Autodesk Inventor part; units mm, degrees
(part 2 of 5)
  line L926 (78.7001, 18.8118) -> (79.4901, 18.8118)
  line L927 (79.4901, 18.8118) -> (79.4901, 18.4118)
  line L928 (78.6251, 11.5368) -> (77.0251, 11.5368)
  line L929 (77.0251, 11.5368) -> (77.0251, 12.1868)
  line L930 (77.0251, 12.1868) -> (78.6251, 12.1868)
  line L931 (78.6251, 12.1868) -> (78.6251, 11.5368)
  line L932 (78.6251, 19.4368) -> (77.0251, 19.4368)
  line L933 (77.0251, 19.4368) -> (77.0251, 20.0868)
  line L934 (77.0251, 20.0868) -> (78.6251, 20.0868)
  line L935 (78.6251, 20.0868) -> (78.6251, 19.4368)
  line L936 (41.1326, 37.3618) -> (41.9226, 37.3618)
  line L937 (41.9226, 37.3618) -> (41.9226, 36.9618)
  line L938 (41.9226, 36.9618) -> (41.1326, 36.9618)
  line L939 (41.1326, 36.9618) -> (41.1326, 37.3618)
  line L940 (38.5926, 37.3618) -> (39.3826, 37.3618)
  line L941 (39.3826, 37.3618) -> (39.3826, 36.9618)
  line L942 (39.3826, 36.9618) -> (38.5926, 36.9618)
  line L943 (38.5926, 36.9618) -> (38.5926, 37.3618)
  line L944 (41.1326, 36.5618) -> (41.9226, 36.5618)
  line L945 (41.9226, 36.5618) -> (41.9226, 36.1618)
  line L946 (41.9226, 36.1618) -> (41.1326, 36.1618)
  line L947 (41.1326, 36.1618) -> (41.1326, 36.5618)
  line L948 (38.5926, 36.5618) -> (39.3826, 36.5618)
  line L949 (39.3826, 36.5618) -> (39.3826, 36.1618)
  line L950 (39.3826, 36.1618) -> (38.5926, 36.1618)
  line L951 (38.5926, 36.1618) -> (38.5926, 36.5618)
  line L952 (41.1326, 35.7618) -> (41.9226, 35.7618)
  line L953 (41.9226, 35.7618) -> (41.9226, 35.3618)
  line L954 (41.9226, 35.3618) -> (41.1326, 35.3618)
  line L955 (41.1326, 35.3618) -> (41.1326, 35.7618)
  line L956 (38.5926, 35.7618) -> (39.3826, 35.7618)
  line L957 (39.3826, 35.7618) -> (39.3826, 35.3618)
  line L958 (39.3826, 35.3618) -> (38.5926, 35.3618)
  line L959 (38.5926, 35.3618) -> (38.5926, 35.7618)
  line L960 (41.1326, 34.9618) -> (41.9226, 34.9618)
  line L961 (41.9226, 34.9618) -> (41.9226, 34.5618)
  line L962 (41.9226, 34.5618) -> (41.1326, 34.5618)
  line L963 (41.1326, 34.5618) -> (41.1326, 34.9618)
  line L964 (38.5926, 34.9618) -> (39.3826, 34.9618)
  line L965 (39.3826, 34.9618) -> (39.3826, 34.5618)
  line L966 (39.3826, 34.5618) -> (38.5926, 34.5618)
  line L967 (38.5926, 34.5618) -> (38.5926, 34.9618)
  line L968 (41.1326, 34.1618) -> (41.9226, 34.1618)
  line L969 (41.9226, 34.1618) -> (41.9226, 33.7618)
  line L970 (41.9226, 33.7618) -> (41.1326, 33.7618)
  line L971 (41.1326, 33.7618) -> (41.1326, 34.1618)
  line L972 (38.5926, 34.1618) -> (39.3826, 34.1618)
  line L973 (39.3826, 34.1618) -> (39.3826, 33.7618)
  line L974 (39.3826, 33.7618) -> (38.5926, 33.7618)
  line L975 (38.5926, 33.7618) -> (38.5926, 34.1618)
  line L976 (41.1326, 33.3618) -> (41.9226, 33.3618)
  line L977 (41.9226, 33.3618) -> (41.9226, 32.9618)
  line L978 (41.9226, 32.9618) -> (41.1326, 32.9618)
  line L979 (41.1326, 32.9618) -> (41.1326, 33.3618)
  line L980 (38.5926, 33.3618) -> (39.3826, 33.3618)
  line L981 (39.3826, 33.3618) -> (39.3826, 32.9618)
  line L982 (39.3826, 32.9618) -> (38.5926, 32.9618)
  line L983 (38.5926, 32.9618) -> (38.5926, 33.3618)
  line L984 (41.1326, 32.5618) -> (41.9226, 32.5618)
  line L985 (41.9226, 32.5618) -> (41.9226, 32.1618)
  line L986 (41.9226, 32.1618) -> (41.1326, 32.1618)
  line L987 (41.1326, 32.1618) -> (41.1326, 32.5618)
  line L988 (38.5926, 32.5618) -> (39.3826, 32.5618)
  line L989 (39.3826, 32.5618) -> (39.3826, 32.1618)
  line L990 (39.3826, 32.1618) -> (38.5926, 32.1618)
  line L991 (38.5926, 32.1618) -> (38.5926, 32.5618)
  line L992 (41.1326, 31.7618) -> (41.9226, 31.7618)
  line L993 (41.9226, 31.7618) -> (41.9226, 31.3618)
  line L994 (41.9226, 31.3618) -> (41.1326, 31.3618)
  line L995 (41.1326, 31.3618) -> (41.1326, 31.7618)
  line L996 (38.5926, 31.7618) -> (39.3826, 31.7618)
  line L997 (39.3826, 31.7618) -> (39.3826, 31.3618)
  line L998 (39.3826, 31.3618) -> (38.5926, 31.3618)
  line L999 (38.5926, 31.3618) -> (38.5926, 31.7618)
  line L1000 (39.4576, 38.6368) -> (41.0576, 38.6368)
  line L1001 (41.0576, 38.6368) -> (41.0576, 37.9868)
  line L1002 (41.0576, 37.9868) -> (39.4576, 37.9868)
  line L1003 (39.4576, 37.9868) -> (39.4576, 38.6368)
  line L1004 (39.4576, 30.7368) -> (41.0576, 30.7368)
  line L1005 (41.0576, 30.7368) -> (41.0576, 30.0868)
  line L1006 (41.0576, 30.0868) -> (39.4576, 30.0868)
  line L1007 (39.4576, 30.0868) -> (39.4576, 30.7368)
  line L1008 (116.3201, 75.0868) -> (117.1101, 75.0868)
  line L1009 (117.1101, 75.0868) -> (117.1101, 74.6868)
  line L1010 (117.1101, 74.6868) -> (116.3201, 74.6868)
  line L1011 (116.3201, 74.6868) -> (116.3201, 75.0868)
  line L1012 (113.7801, 75.0868) -> (114.5701, 75.0868)
  line L1013 (114.5701, 75.0868) -> (114.5701, 74.6868)
  line L1014 (114.5701, 74.6868) -> (113.7801, 74.6868)
  line L1015 (113.7801, 74.6868) -> (113.7801, 75.0868)
  line L1016 (116.3201, 74.2868) -> (117.1101, 74.2868)
  line L1017 (117.1101, 74.2868) -> (117.1101, 73.8868)
  line L1018 (117.1101, 73.8868) -> (116.3201, 73.8868)
  line L1019 (116.3201, 73.8868) -> (116.3201, 74.2868)
  line L1020 (113.7801, 74.2868) -> (114.5701, 74.2868)
  line L1021 (114.5701, 74.2868) -> (114.5701, 73.8868)
  line L1022 (114.5701, 73.8868) -> (113.7801, 73.8868)
  line L1023 (113.7801, 73.8868) -> (113.7801, 74.2868)
  line L1024 (116.3201, 73.4868) -> (117.1101, 73.4868)
  line L1025 (117.1101, 73.4868) -> (117.1101, 73.0868)
  line L1026 (117.1101, 73.0868) -> (116.3201, 73.0868)
  line L1027 (116.3201, 73.0868) -> (116.3201, 73.4868)
  line L1028 (113.7801, 73.4868) -> (114.5701, 73.4868)
  line L1029 (114.5701, 73.4868) -> (114.5701, 73.0868)
  line L1030 (114.5701, 73.0868) -> (113.7801, 73.0868)
  line L1031 (113.7801, 73.0868) -> (113.7801, 73.4868)
  line L1032 (116.3201, 72.6868) -> (117.1101, 72.6868)
  line L1033 (117.1101, 72.6868) -> (117.1101, 72.2868)
  line L1034 (117.1101, 72.2868) -> (116.3201, 72.2868)
  line L1035 (116.3201, 72.2868) -> (116.3201, 72.6868)
  line L1036 (113.7801, 72.6868) -> (114.5701, 72.6868)
  line L1037 (114.5701, 72.6868) -> (114.5701, 72.2868)
  line L1038 (114.5701, 72.2868) -> (113.7801, 72.2868)
  line L1039 (113.7801, 72.2868) -> (113.7801, 72.6868)
  line L1040 (116.3201, 71.8868) -> (117.1101, 71.8868)
  line L1041 (117.1101, 71.8868) -> (117.1101, 71.4868)
  line L1042 (117.1101, 71.4868) -> (116.3201, 71.4868)
  line L1043 (116.3201, 71.4868) -> (116.3201, 71.8868)
  line L1044 (113.7801, 71.8868) -> (114.5701, 71.8868)
  line L1045 (114.5701, 71.8868) -> (114.5701, 71.4868)
  line L1046 (114.5701, 71.4868) -> (113.7801, 71.4868)
  line L1047 (113.7801, 71.4868) -> (113.7801, 71.8868)
  line L1048 (116.3201, 71.0868) -> (117.1101, 71.0868)
  line L1049 (117.1101, 71.0868) -> (117.1101, 70.6868)
  line L1050 (117.1101, 70.6868) -> (116.3201, 70.6868)
  line L1051 (116.3201, 70.6868) -> (116.3201, 71.0868)
  line L1052 (113.7801, 71.0868) -> (114.5701, 71.0868)
  line L1053 (114.5701, 71.0868) -> (114.5701, 70.6868)
  line L1054 (114.5701, 70.6868) -> (113.7801, 70.6868)
  line L1055 (113.7801, 70.6868) -> (113.7801, 71.0868)
  line L1056 (116.3201, 70.2868) -> (117.1101, 70.2868)
  line L1057 (117.1101, 70.2868) -> (117.1101, 69.8868)
  line L1058 (117.1101, 69.8868) -> (116.3201, 69.8868)
  line L1059 (116.3201, 69.8868) -> (116.3201, 70.2868)
  line L1060 (113.7801, 70.2868) -> (114.5701, 70.2868)
  line L1061 (114.5701, 70.2868) -> (114.5701, 69.8868)
  line L1062 (114.5701, 69.8868) -> (113.7801, 69.8868)
  line L1063 (113.7801, 69.8868) -> (113.7801, 70.2868)
  line L1064 (116.3201, 69.4868) -> (117.1101, 69.4868)
  line L1065 (117.1101, 69.4868) -> (117.1101, 69.0868)
  line L1066 (117.1101, 69.0868) -> (116.3201, 69.0868)
  line L1067 (116.3201, 69.0868) -> (116.3201, 69.4868)
  line L1068 (113.7801, 69.4868) -> (114.5701, 69.4868)
  line L1069 (114.5701, 69.4868) -> (114.5701, 69.0868)
  line L1070 (114.5701, 69.0868) -> (113.7801, 69.0868)
  line L1071 (113.7801, 69.0868) -> (113.7801, 69.4868)
  line L1072 (114.6451, 76.3618) -> (116.2451, 76.3618)
  line L1073 (116.2451, 76.3618) -> (116.2451, 75.7118)
  line L1074 (116.2451, 75.7118) -> (114.6451, 75.7118)
  line L1075 (114.6451, 75.7118) -> (114.6451, 76.3618)
  line L1076 (114.6451, 68.4618) -> (116.2451, 68.4618)
  line L1077 (116.2451, 68.4618) -> (116.2451, 67.8118)
  line L1078 (116.2451, 67.8118) -> (114.6451, 67.8118)
  line L1079 (114.6451, 67.8118) -> (114.6451, 68.4618)
  line L1080 (97.5651, 75.1118) -> (98.3551, 75.1118)
  line L1081 (98.3551, 75.1118) -> (98.3551, 74.7118)
  line L1082 (98.3551, 74.7118) -> (97.5651, 74.7118)
  line L1083 (97.5651, 74.7118) -> (97.5651, 75.1118)
  line L1084 (95.0251, 75.1118) -> (95.8151, 75.1118)
  line L1085 (95.8151, 75.1118) -> (95.8151, 74.7118)
  line L1086 (95.8151, 74.7118) -> (95.0251, 74.7118)
  line L1087 (95.0251, 74.7118) -> (95.0251, 75.1118)
  line L1088 (97.5651, 74.3118) -> (98.3551, 74.3118)
  line L1089 (98.3551, 74.3118) -> (98.3551, 73.9118)
  line L1090 (98.3551, 73.9118) -> (97.5651, 73.9118)
  line L1091 (97.5651, 73.9118) -> (97.5651, 74.3118)
  line L1092 (95.0251, 74.3118) -> (95.8151, 74.3118)
  line L1093 (95.8151, 74.3118) -> (95.8151, 73.9118)
  line L1094 (95.8151, 73.9118) -> (95.0251, 73.9118)
  line L1095 (95.0251, 73.9118) -> (95.0251, 74.3118)
  line L1096 (97.5651, 73.5118) -> (98.3551, 73.5118)
  line L1097 (98.3551, 73.5118) -> (98.3551, 73.1118)
  line L1098 (98.3551, 73.1118) -> (97.5651, 73.1118)
  line L1099 (97.5651, 73.1118) -> (97.5651, 73.5118)
  line L1100 (95.0251, 73.5118) -> (95.8151, 73.5118)
  line L1101 (95.8151, 73.5118) -> (95.8151, 73.1118)
  line L1102 (95.8151, 73.1118) -> (95.0251, 73.1118)
  line L1103 (95.0251, 73.1118) -> (95.0251, 73.5118)
  line L1104 (97.5651, 72.7118) -> (98.3551, 72.7118)
  line L1105 (98.3551, 72.7118) -> (98.3551, 72.3118)
  line L1106 (98.3551, 72.3118) -> (97.5651, 72.3118)
  line L1107 (97.5651, 72.3118) -> (97.5651, 72.7118)
  line L1108 (95.0251, 72.7118) -> (95.8151, 72.7118)
  line L1109 (95.8151, 72.7118) -> (95.8151, 72.3118)
  line L1110 (95.8151, 72.3118) -> (95.0251, 72.3118)
  line L1111 (95.0251, 72.3118) -> (95.0251, 72.7118)
  line L1112 (97.5651, 71.9118) -> (98.3551, 71.9118)
  line L1113 (98.3551, 71.9118) -> (98.3551, 71.5118)
  line L1114 (98.3551, 71.5118) -> (97.5651, 71.5118)
  line L1115 (97.5651, 71.5118) -> (97.5651, 71.9118)
  line L1116 (95.0251, 71.9118) -> (95.8151, 71.9118)
  line L1117 (95.8151, 71.9118) -> (95.8151, 71.5118)
  line L1118 (95.8151, 71.5118) -> (95.0251, 71.5118)
  line L1119 (95.0251, 71.5118) -> (95.0251, 71.9118)
  line L1120 (97.5651, 71.1118) -> (98.3551, 71.1118)
  line L1121 (98.3551, 71.1118) -> (98.3551, 70.7118)
  line L1122 (98.3551, 70.7118) -> (97.5651, 70.7118)
  line L1123 (97.5651, 70.7118) -> (97.5651, 71.1118)
  line L1124 (95.0251, 71.1118) -> (95.8151, 71.1118)
  line L1125 (95.8151, 71.1118) -> (95.8151, 70.7118)
  line L1126 (95.8151, 70.7118) -> (95.0251, 70.7118)
  line L1127 (95.0251, 70.7118) -> (95.0251, 71.1118)
  line L1128 (97.5651, 70.3118) -> (98.3551, 70.3118)
  line L1129 (98.3551, 70.3118) -> (98.3551, 69.9118)
  line L1130 (98.3551, 69.9118) -> (97.5651, 69.9118)
  line L1131 (97.5651, 69.9118) -> (97.5651, 70.3118)
  line L1132 (95.0251, 70.3118) -> (95.8151, 70.3118)
  line L1133 (95.8151, 70.3118) -> (95.8151, 69.9118)
  line L1134 (95.8151, 69.9118) -> (95.0251, 69.9118)
  line L1135 (95.0251, 69.9118) -> (95.0251, 70.3118)
  line L1136 (97.5651, 69.5118) -> (98.3551, 69.5118)
  line L1137 (98.3551, 69.5118) -> (98.3551, 69.1118)
  line L1138 (98.3551, 69.1118) -> (97.5651, 69.1118)
  line L1139 (97.5651, 69.1118) -> (97.5651, 69.5118)
  line L1140 (95.0251, 69.5118) -> (95.8151, 69.5118)
  line L1141 (95.8151, 69.5118) -> (95.8151, 69.1118)
  line L1142 (95.8151, 69.1118) -> (95.0251, 69.1118)
  line L1143 (95.0251, 69.1118) -> (95.0251, 69.5118)
  line L1144 (95.8901, 76.3868) -> (97.4901, 76.3868)
  line L1145 (97.4901, 76.3868) -> (97.4901, 75.7368)
  line L1146 (97.4901, 75.7368) -> (95.8901, 75.7368)
  line L1147 (95.8901, 75.7368) -> (95.8901, 76.3868)
  line L1148 (95.8901, 68.4868) -> (97.4901, 68.4868)
  line L1149 (97.4901, 68.4868) -> (97.4901, 67.8368)
  line L1150 (97.4901, 67.8368) -> (95.8901, 67.8368)
  line L1151 (95.8901, 67.8368) -> (95.8901, 68.4868)
  line L1152 (114.6676, 50.3618) -> (113.8776, 50.3618)
  line L1153 (113.8776, 50.3618) -> (113.8776, 50.7618)
  line L1154 (113.8776, 50.7618) -> (114.6676, 50.7618)
  line L1155 (114.6676, 50.7618) -> (114.6676, 50.3618)
  line L1156 (117.2076, 50.3618) -> (116.4176, 50.3618)
  line L1157 (116.4176, 50.3618) -> (116.4176, 50.7618)
  line L1158 (116.4176, 50.7618) -> (117.2076, 50.7618)
  line L1159 (117.2076, 50.7618) -> (117.2076, 50.3618)
  line L1160 (114.6676, 51.1618) -> (113.8776, 51.1618)
  line L1161 (113.8776, 51.1618) -> (113.8776, 51.5618)
  line L1162 (113.8776, 51.5618) -> (114.6676, 51.5618)
  line L1163 (114.6676, 51.5618) -> (114.6676, 51.1618)
  line L1164 (117.2076, 51.1618) -> (116.4176, 51.1618)
  line L1165 (116.4176, 51.1618) -> (116.4176, 51.5618)
  line L1166 (116.4176, 51.5618) -> (117.2076, 51.5618)
  line L1167 (117.2076, 51.5618) -> (117.2076, 51.1618)
  line L1168 (114.6676, 51.9618) -> (113.8776, 51.9618)
  line L1169 (113.8776, 51.9618) -> (113.8776, 52.3618)
  line L1170 (113.8776, 52.3618) -> (114.6676, 52.3618)
  line L1171 (114.6676, 52.3618) -> (114.6676, 51.9618)
  line L1172 (117.2076, 51.9618) -> (116.4176, 51.9618)
  line L1173 (116.4176, 51.9618) -> (116.4176, 52.3618)
  line L1174 (116.4176, 52.3618) -> (117.2076, 52.3618)
  line L1175 (117.2076, 52.3618) -> (117.2076, 51.9618)
  line L1176 (114.6676, 52.7618) -> (113.8776, 52.7618)
  line L1177 (113.8776, 52.7618) -> (113.8776, 53.1618)
  line L1178 (113.8776, 53.1618) -> (114.6676, 53.1618)
  line L1179 (114.6676, 53.1618) -> (114.6676, 52.7618)
  line L1180 (117.2076, 52.7618) -> (116.4176, 52.7618)
  line L1181 (116.4176, 52.7618) -> (116.4176, 53.1618)
  line L1182 (116.4176, 53.1618) -> (117.2076, 53.1618)
  line L1183 (117.2076, 53.1618) -> (117.2076, 52.7618)
  line L1184 (114.6676, 53.5618) -> (113.8776, 53.5618)
  line L1185 (113.8776, 53.5618) -> (113.8776, 53.9618)
  line L1186 (113.8776, 53.9618) -> (114.6676, 53.9618)
  line L1187 (114.6676, 53.9618) -> (114.6676, 53.5618)
  line L1188 (117.2076, 53.5618) -> (116.4176, 53.5618)
  line L1189 (116.4176, 53.5618) -> (116.4176, 53.9618)
  line L1190 (116.4176, 53.9618) -> (117.2076, 53.9618)
  line L1191 (117.2076, 53.9618) -> (117.2076, 53.5618)
  line L1192 (114.6676, 54.3618) -> (113.8776, 54.3618)
  line L1193 (113.8776, 54.3618) -> (113.8776, 54.7618)
  line L1194 (113.8776, 54.7618) -> (114.6676, 54.7618)
  line L1195 (114.6676, 54.7618) -> (114.6676, 54.3618)
  line L1196 (117.2076, 54.3618) -> (116.4176, 54.3618)
  line L1197 (116.4176, 54.3618) -> (116.4176, 54.7618)
  line L1198 (116.4176, 54.7618) -> (117.2076, 54.7618)
  line L1199 (117.2076, 54.7618) -> (117.2076, 54.3618)
  line L1200 (114.6676, 55.1618) -> (113.8776, 55.1618)
  line L1201 (113.8776, 55.1618) -> (113.8776, 55.5618)
  line L1202 (113.8776, 55.5618) -> (114.6676, 55.5618)
  line L1203 (114.6676, 55.5618) -> (114.6676, 55.1618)
  line L1204 (117.2076, 55.1618) -> (116.4176, 55.1618)
  line L1205 (116.4176, 55.1618) -> (116.4176, 55.5618)
  line L1206 (116.4176, 55.5618) -> (117.2076, 55.5618)
  line L1207 (117.2076, 55.5618) -> (117.2076, 55.1618)
  line L1208 (114.6676, 55.9618) -> (113.8776, 55.9618)
  line L1209 (113.8776, 55.9618) -> (113.8776, 56.3618)
  line L1210 (113.8776, 56.3618) -> (114.6676, 56.3618)
  line L1211 (114.6676, 56.3618) -> (114.6676, 55.9618)
  line L1212 (117.2076, 55.9618) -> (116.4176, 55.9618)
  line L1213 (116.4176, 55.9618) -> (116.4176, 56.3618)
  line L1214 (116.4176, 56.3618) -> (117.2076, 56.3618)
  line L1215 (117.2076, 56.3618) -> (117.2076, 55.9618)
  line L1216 (116.3426, 49.0868) -> (114.7426, 49.0868)
  line L1217 (114.7426, 49.0868) -> (114.7426, 49.7368)
  line L1218 (114.7426, 49.7368) -> (116.3426, 49.7368)
  line L1219 (116.3426, 49.7368) -> (116.3426, 49.0868)
  line L1220 (116.3426, 56.9868) -> (114.7426, 56.9868)
  line L1221 (114.7426, 56.9868) -> (114.7426, 57.6368)
  line L1222 (114.7426, 57.6368) -> (116.3426, 57.6368)
  line L1223 (116.3426, 57.6368) -> (116.3426, 56.9868)
  line L1224 (57.9176, 50.4868) -> (57.1276, 50.4868)
  line L1225 (57.1276, 50.4868) -> (57.1276, 50.8868)
  line L1226 (57.1276, 50.8868) -> (57.9176, 50.8868)
  line L1227 (57.9176, 50.8868) -> (57.9176, 50.4868)
  line L1228 (60.4576, 50.4868) -> (59.6676, 50.4868)
  line L1229 (59.6676, 50.4868) -> (59.6676, 50.8868)
  line L1230 (59.6676, 50.8868) -> (60.4576, 50.8868)
  line L1231 (60.4576, 50.8868) -> (60.4576, 50.4868)
  line L1232 (57.9176, 51.2868) -> (57.1276, 51.2868)
  line L1233 (57.1276, 51.2868) -> (57.1276, 51.6868)
  line L1234 (57.1276, 51.6868) -> (57.9176, 51.6868)
  line L1235 (57.9176, 51.6868) -> (57.9176, 51.2868)
  line L1236 (60.4576, 51.2868) -> (59.6676, 51.2868)
  line L1237 (59.6676, 51.2868) -> (59.6676, 51.6868)
  line L1238 (59.6676, 51.6868) -> (60.4576, 51.6868)
  line L1239 (60.4576, 51.6868) -> (60.4576, 51.2868)
  line L1240 (57.9176, 52.0868) -> (57.1276, 52.0868)
  line L1241 (57.1276, 52.0868) -> (57.1276, 52.4868)
  line L1242 (57.1276, 52.4868) -> (57.9176, 52.4868)
  line L1243 (57.9176, 52.4868) -> (57.9176, 52.0868)
  line L1244 (60.4576, 52.0868) -> (59.6676, 52.0868)
  line L1245 (59.6676, 52.0868) -> (59.6676, 52.4868)
  line L1246 (59.6676, 52.4868) -> (60.4576, 52.4868)
  line L1247 (60.4576, 52.4868) -> (60.4576, 52.0868)
  line L1248 (57.9176, 52.8868) -> (57.1276, 52.8868)
  line L1249 (57.1276, 52.8868) -> (57.1276, 53.2868)
  line L1250 (57.1276, 53.2868) -> (57.9176, 53.2868)
  line L1251 (57.9176, 53.2868) -> (57.9176, 52.8868)
  line L1252 (60.4576, 52.8868) -> (59.6676, 52.8868)
  line L1253 (59.6676, 52.8868) -> (59.6676, 53.2868)
  line L1254 (59.6676, 53.2868) -> (60.4576, 53.2868)
  line L1255 (60.4576, 53.2868) -> (60.4576, 52.8868)
  line L1256 (57.9176, 53.6868) -> (57.1276, 53.6868)
  line L1257 (57.1276, 53.6868) -> (57.1276, 54.0868)
  line L1258 (57.1276, 54.0868) -> (57.9176, 54.0868)
  line L1259 (57.9176, 54.0868) -> (57.9176, 53.6868)
  line L1260 (60.4576, 53.6868) -> (59.6676, 53.6868)
  line L1261 (59.6676, 53.6868) -> (59.6676, 54.0868)
  line L1262 (59.6676, 54.0868) -> (60.4576, 54.0868)
  line L1263 (60.4576, 54.0868) -> (60.4576, 53.6868)
  line L1264 (57.9176, 54.4868) -> (57.1276, 54.4868)
  line L1265 (57.1276, 54.4868) -> (57.1276, 54.8868)
  line L1266 (57.1276, 54.8868) -> (57.9176, 54.8868)
  line L1267 (57.9176, 54.8868) -> (57.9176, 54.4868)
  line L1268 (60.4576, 54.4868) -> (59.6676, 54.4868)
  line L1269 (59.6676, 54.4868) -> (59.6676, 54.8868)
  line L1270 (59.6676, 54.8868) -> (60.4576, 54.8868)
  line L1271 (60.4576, 54.8868) -> (60.4576, 54.4868)
  line L1272 (57.9176, 55.2868) -> (57.1276, 55.2868)
  line L1273 (57.1276, 55.2868) -> (57.1276, 55.6868)
  line L1274 (57.1276, 55.6868) -> (57.9176, 55.6868)
  line L1275 (57.9176, 55.6868) -> (57.9176, 55.2868)
  line L1276 (60.4576, 55.2868) -> (59.6676, 55.2868)
  line L1277 (59.6676, 55.2868) -> (59.6676, 55.6868)
  line L1278 (59.6676, 55.6868) -> (60.4576, 55.6868)
  line L1279 (60.4576, 55.6868) -> (60.4576, 55.2868)
  line L1280 (57.9176, 56.0868) -> (57.1276, 56.0868)
  line L1281 (57.1276, 56.0868) -> (57.1276, 56.4868)
  line L1282 (57.1276, 56.4868) -> (57.9176, 56.4868)
  line L1283 (57.9176, 56.4868) -> (57.9176, 56.0868)
  line L1284 (60.4576, 56.0868) -> (59.6676, 56.0868)
  line L1285 (59.6676, 56.0868) -> (59.6676, 56.4868)
  line L1286 (59.6676, 56.4868) -> (60.4576, 56.4868)
  line L1287 (60.4576, 56.4868) -> (60.4576, 56.0868)
  line L1288 (59.5926, 49.2118) -> (57.9926, 49.2118)
  line L1289 (57.9926, 49.2118) -> (57.9926, 49.8618)
  line L1290 (57.9926, 49.8618) -> (59.5926, 49.8618)
  line L1291 (59.5926, 49.8618) -> (59.5926, 49.2118)
  line L1292 (59.5926, 57.1118) -> (57.9926, 57.1118)
  line L1293 (57.9926, 57.1118) -> (57.9926, 57.7618)
  line L1294 (57.9926, 57.7618) -> (59.5926, 57.7618)
  line L1295 (59.5926, 57.7618) -> (59.5926, 57.1118)
  line L1296 (41.0576, 75.1368) -> (41.8476, 75.1368)
  line L1297 (41.8476, 75.1368) -> (41.8476, 74.7368)
  line L1298 (41.8476, 74.7368) -> (41.0576, 74.7368)
  line L1299 (41.0576, 74.7368) -> (41.0576, 75.1368)
  line L1300 (38.5176, 75.1368) -> (39.3076, 75.1368)
  line L1301 (39.3076, 75.1368) -> (39.3076, 74.7368)
  line L1302 (39.3076, 74.7368) -> (38.5176, 74.7368)
  line L1303 (38.5176, 74.7368) -> (38.5176, 75.1368)
  line L1304 (41.0576, 74.3368) -> (41.8476, 74.3368)
  line L1305 (41.8476, 74.3368) -> (41.8476, 73.9368)
  line L1306 (41.8476, 73.9368) -> (41.0576, 73.9368)
  line L1307 (41.0576, 73.9368) -> (41.0576, 74.3368)
  line L1308 (38.5176, 74.3368) -> (39.3076, 74.3368)
  line L1309 (39.3076, 74.3368) -> (39.3076, 73.9368)
  line L1310 (39.3076, 73.9368) -> (38.5176, 73.9368)
  line L1311 (38.5176, 73.9368) -> (38.5176, 74.3368)
  line L1312 (41.0576, 73.5368) -> (41.8476, 73.5368)
  line L1313 (41.8476, 73.5368) -> (41.8476, 73.1368)
  line L1314 (41.8476, 73.1368) -> (41.0576, 73.1368)
  line L1315 (41.0576, 73.1368) -> (41.0576, 73.5368)
  line L1316 (38.5176, 73.5368) -> (39.3076, 73.5368)
  line L1317 (39.3076, 73.5368) -> (39.3076, 73.1368)
  line L1318 (39.3076, 73.1368) -> (38.5176, 73.1368)
  line L1319 (38.5176, 73.1368) -> (38.5176, 73.5368)
  line L1320 (41.0576, 72.7368) -> (41.8476, 72.7368)
  line L1321 (41.8476, 72.7368) -> (41.8476, 72.3368)
  line L1322 (41.8476, 72.3368) -> (41.0576, 72.3368)
  line L1323 (41.0576, 72.3368) -> (41.0576, 72.7368)
  line L1324 (38.5176, 72.7368) -> (39.3076, 72.7368)
  line L1325 (39.3076, 72.7368) -> (39.3076, 72.3368)
  line L1326 (39.3076, 72.3368) -> (38.5176, 72.3368)
  line L1327 (38.5176, 72.3368) -> (38.5176, 72.7368)
  line L1328 (41.0576, 71.9368) -> (41.8476, 71.9368)
  line L1329 (41.8476, 71.9368) -> (41.8476, 71.5368)
  line L1330 (41.8476, 71.5368) -> (41.0576, 71.5368)
  line L1331 (41.0576, 71.5368) -> (41.0576, 71.9368)
  line L1332 (38.5176, 71.9368) -> (39.3076, 71.9368)
  line L1333 (39.3076, 71.9368) -> (39.3076, 71.5368)
  line L1334 (39.3076, 71.5368) -> (38.5176, 71.5368)
  line L1335 (38.5176, 71.5368) -> (38.5176, 71.9368)
  line L1336 (41.0576, 71.1368) -> (41.8476, 71.1368)
  line L1337 (41.8476, 71.1368) -> (41.8476, 70.7368)
  line L1338 (41.8476, 70.7368) -> (41.0576, 70.7368)
  line L1339 (41.0576, 70.7368) -> (41.0576, 71.1368)
  line L1340 (38.5176, 71.1368) -> (39.3076, 71.1368)
  line L1341 (39.3076, 71.1368) -> (39.3076, 70.7368)
  line L1342 (39.3076, 70.7368) -> (38.5176, 70.7368)
  line L1343 (38.5176, 70.7368) -> (38.5176, 71.1368)
  line L1344 (41.0576, 70.3368) -> (41.8476, 70.3368)
  line L1345 (41.8476, 70.3368) -> (41.8476, 69.9368)
  line L1346 (41.8476, 69.9368) -> (41.0576, 69.9368)
  line L1347 (41.0576, 69.9368) -> (41.0576, 70.3368)
  line L1348 (38.5176, 70.3368) -> (39.3076, 70.3368)
  line L1349 (39.3076, 70.3368) -> (39.3076, 69.9368)
  line L1350 (39.3076, 69.9368) -> (38.5176, 69.9368)
  line L1351 (38.5176, 69.9368) -> (38.5176, 70.3368)
  line L1352 (41.0576, 69.5368) -> (41.8476, 69.5368)
  line L1353 (41.8476, 69.5368) -> (41.8476, 69.1368)
  line L1354 (41.8476, 69.1368) -> (41.0576, 69.1368)
  line L1355 (41.0576, 69.1368) -> (41.0576, 69.5368)
  line L1356 (38.5176, 69.5368) -> (39.3076, 69.5368)
  line L1357 (39.3076, 69.5368) -> (39.3076, 69.1368)
  line L1358 (39.3076, 69.1368) -> (38.5176, 69.1368)
  line L1359 (38.5176, 69.1368) -> (38.5176, 69.5368)
  line L1360 (39.3826, 76.4118) -> (40.9826, 76.4118)
  line L1361 (40.9826, 76.4118) -> (40.9826, 75.7618)
  line L1362 (40.9826, 75.7618) -> (39.3826, 75.7618)
  line L1363 (39.3826, 75.7618) -> (39.3826, 76.4118)
  line L1364 (39.3826, 68.5118) -> (40.9826, 68.5118)
  line L1365 (40.9826, 68.5118) -> (40.9826, 67.8618)
  line L1366 (40.9826, 67.8618) -> (39.3826, 67.8618)
  line L1367 (39.3826, 67.8618) -> (39.3826, 68.5118)
  line L1368 (20.3551, 50.4368) -> (19.5651, 50.4368)
  line L1369 (19.5651, 50.4368) -> (19.5651, 50.8368)
  line L1370 (19.5651, 50.8368) -> (20.3551, 50.8368)
  line L1371 (20.3551, 50.8368) -> (20.3551, 50.4368)
  line L1372 (22.8951, 50.4368) -> (22.1051, 50.4368)
  line L1373 (22.1051, 50.4368) -> (22.1051, 50.8368)
  line L1374 (22.1051, 50.8368) -> (22.8951, 50.8368)
  line L1375 (22.8951, 50.8368) -> (22.8951, 50.4368)
  line L1376 (20.3551, 51.2368) -> (19.5651, 51.2368)
  line L1377 (19.5651, 51.2368) -> (19.5651, 51.6368)
  line L1378 (19.5651, 51.6368) -> (20.3551, 51.6368)
  line L1379 (20.3551, 51.6368) -> (20.3551, 51.2368)
  line L1380 (22.8951, 51.2368) -> (22.1051, 51.2368)
  line L1381 (22.1051, 51.2368) -> (22.1051, 51.6368)
  line L1382 (22.1051, 51.6368) -> (22.8951, 51.6368)
  line L1383 (22.8951, 51.6368) -> (22.8951, 51.2368)
  line L1384 (20.3551, 52.0368) -> (19.5651, 52.0368)
  line L1385 (19.5651, 52.0368) -> (19.5651, 52.4368)
  line L1386 (19.5651, 52.4368) -> (20.3551, 52.4368)
  line L1387 (20.3551, 52.4368) -> (20.3551, 52.0368)
  line L1388 (22.8951, 52.0368) -> (22.1051, 52.0368)
  line L1389 (22.1051, 52.0368) -> (22.1051, 52.4368)
  line L1390 (22.1051, 52.4368) -> (22.8951, 52.4368)
  line L1391 (22.8951, 52.4368) -> (22.8951, 52.0368)
  line L1392 (20.3551, 52.8368) -> (19.5651, 52.8368)
  line L1393 (19.5651, 52.8368) -> (19.5651, 53.2368)
  line L1394 (19.5651, 53.2368) -> (20.3551, 53.2368)
  line L1395 (20.3551, 53.2368) -> (20.3551, 52.8368)
  line L1396 (22.8951, 52.8368) -> (22.1051, 52.8368)
  line L1397 (22.1051, 52.8368) -> (22.1051, 53.2368)
  line L1398 (22.1051, 53.2368) -> (22.8951, 53.2368)
  line L1399 (22.8951, 53.2368) -> (22.8951, 52.8368)
  line L1400 (20.3551, 53.6368) -> (19.5651, 53.6368)
  line L1401 (19.5651, 53.6368) -> (19.5651, 54.0368)
  line L1402 (19.5651, 54.0368) -> (20.3551, 54.0368)
  line L1403 (20.3551, 54.0368) -> (20.3551, 53.6368)
  line L1404 (22.8951, 53.6368) -> (22.1051, 53.6368)
  line L1405 (22.1051, 53.6368) -> (22.1051, 54.0368)
  line L1406 (22.1051, 54.0368) -> (22.8951, 54.0368)
  line L1407 (22.8951, 54.0368) -> (22.8951, 53.6368)
  line L1408 (20.3551, 54.4368) -> (19.5651, 54.4368)
  line L1409 (19.5651, 54.4368) -> (19.5651, 54.8368)
  line L1410 (19.5651, 54.8368) -> (20.3551, 54.8368)
  line L1411 (20.3551, 54.8368) -> (20.3551, 54.4368)
  line L1412 (22.8951, 54.4368) -> (22.1051, 54.4368)
  line L1413 (22.1051, 54.4368) -> (22.1051, 54.8368)
  line L1414 (22.1051, 54.8368) -> (22.8951, 54.8368)
  line L1415 (22.8951, 54.8368) -> (22.8951, 54.4368)
  line L1416 (20.3551, 55.2368) -> (19.5651, 55.2368)
  line L1417 (19.5651, 55.2368) -> (19.5651, 55.6368)
  line L1418 (19.5651, 55.6368) -> (20.3551, 55.6368)
  line L1419 (20.3551, 55.6368) -> (20.3551, 55.2368)
  line L1420 (22.8951, 55.2368) -> (22.1051, 55.2368)
  line L1421 (22.1051, 55.2368) -> (22.1051, 55.6368)
  line L1422 (22.1051, 55.6368) -> (22.8951, 55.6368)
  line L1423 (22.8951, 55.6368) -> (22.8951, 55.2368)
  line L1424 (20.3551, 56.0368) -> (19.5651, 56.0368)
  line L1425 (19.5651, 56.0368) -> (19.5651, 56.4368)
  line L1426 (19.5651, 56.4368) -> (20.3551, 56.4368)
  line L1427 (20.3551, 56.4368) -> (20.3551, 56.0368)
  line L1428 (22.8951, 56.0368) -> (22.1051, 56.0368)
  line L1429 (22.1051, 56.0368) -> (22.1051, 56.4368)
  line L1430 (22.1051, 56.4368) -> (22.8951, 56.4368)
  line L1431 (22.8951, 56.4368) -> (22.8951, 56.0368)
  line L1432 (22.0301, 49.1618) -> (20.4301, 49.1618)
  line L1433 (20.4301, 49.1618) -> (20.4301, 49.8118)
  line L1434 (20.4301, 49.8118) -> (22.0301, 49.8118)
  line L1435 (22.0301, 49.8118) -> (22.0301, 49.1618)
  line L1436 (22.0301, 57.0618) -> (20.4301, 57.0618)
  line L1437 (20.4301, 57.0618) -> (20.4301, 57.7118)
  line L1438 (20.4301, 57.7118) -> (22.0301, 57.7118)
  line L1439 (22.0301, 57.7118) -> (22.0301, 57.0618)
  line L1440 (59.9576, 37.2618) -> (60.7476, 37.2618)
  line L1441 (60.7476, 37.2618) -> (60.7476, 36.8618)
  line L1442 (60.7476, 36.8618) -> (59.9576, 36.8618)
  line L1443 (59.9576, 36.8618) -> (59.9576, 37.2618)
  line L1444 (57.4176, 37.2618) -> (58.2076, 37.2618)
  line L1445 (58.2076, 37.2618) -> (58.2076, 36.8618)
  line L1446 (58.2076, 36.8618) -> (57.4176, 36.8618)
  line L1447 (57.4176, 36.8618) -> (57.4176, 37.2618)
  line L1448 (59.9576, 36.4618) -> (60.7476, 36.4618)
  line L1449 (60.7476, 36.4618) -> (60.7476, 36.0618)
  line L1450 (60.7476, 36.0618) -> (59.9576, 36.0618)
  line L1451 (59.9576, 36.0618) -> (59.9576, 36.4618)
  line L1452 (57.4176, 36.4618) -> (58.2076, 36.4618)
  line L1453 (58.2076, 36.4618) -> (58.2076, 36.0618)
  line L1454 (58.2076, 36.0618) -> (57.4176, 36.0618)
  line L1455 (57.4176, 36.0618) -> (57.4176, 36.4618)
  line L1456 (59.9576, 35.6618) -> (60.7476, 35.6618)
  line L1457 (60.7476, 35.6618) -> (60.7476, 35.2618)
  line L1458 (60.7476, 35.2618) -> (59.9576, 35.2618)
  line L1459 (59.9576, 35.2618) -> (59.9576, 35.6618)
  line L1460 (57.4176, 35.6618) -> (58.2076, 35.6618)
  line L1461 (58.2076, 35.6618) -> (58.2076, 35.2618)
  line L1462 (58.2076, 35.2618) -> (57.4176, 35.2618)
  line L1463 (57.4176, 35.2618) -> (57.4176, 35.6618)
  line L1464 (59.9576, 34.8618) -> (60.7476, 34.8618)
  line L1465 (60.7476, 34.8618) -> (60.7476, 34.4618)
  line L1466 (60.7476, 34.4618) -> (59.9576, 34.4618)
  line L1467 (59.9576, 34.4618) -> (59.9576, 34.8618)
  line L1468 (57.4176, 34.8618) -> (58.2076, 34.8618)
  line L1469 (58.2076, 34.8618) -> (58.2076, 34.4618)
  line L1470 (58.2076, 34.4618) -> (57.4176, 34.4618)
  line L1471 (57.4176, 34.4618) -> (57.4176, 34.8618)
  line L1472 (59.9576, 34.0618) -> (60.7476, 34.0618)
  line L1473 (60.7476, 34.0618) -> (60.7476, 33.6618)
  line L1474 (60.7476, 33.6618) -> (59.9576, 33.6618)
  line L1475 (59.9576, 33.6618) -> (59.9576, 34.0618)
  line L1476 (57.4176, 34.0618) -> (58.2076, 34.0618)
  line L1477 (58.2076, 34.0618) -> (58.2076, 33.6618)
  line L1478 (58.2076, 33.6618) -> (57.4176, 33.6618)
  line L1479 (57.4176, 33.6618) -> (57.4176, 34.0618)
  line L1480 (59.9576, 33.2618) -> (60.7476, 33.2618)
  line L1481 (60.7476, 33.2618) -> (60.7476, 32.8618)
  line L1482 (60.7476, 32.8618) -> (59.9576, 32.8618)
  line L1483 (59.9576, 32.8618) -> (59.9576, 33.2618)
  line L1484 (57.4176, 33.2618) -> (58.2076, 33.2618)
  line L1485 (58.2076, 33.2618) -> (58.2076, 32.8618)
  line L1486 (58.2076, 32.8618) -> (57.4176, 32.8618)
  line L1487 (57.4176, 32.8618) -> (57.4176, 33.2618)
  line L1488 (59.9576, 32.4618) -> (60.7476, 32.4618)
  line L1489 (60.7476, 32.4618) -> (60.7476, 32.0618)
  line L1490 (60.7476, 32.0618) -> (59.9576, 32.0618)
  line L1491 (59.9576, 32.0618) -> (59.9576, 32.4618)
  line L1492 (57.4176, 32.4618) -> (58.2076, 32.4618)
  line L1493 (58.2076, 32.4618) -> (58.2076, 32.0618)
  line L1494 (58.2076, 32.0618) -> (57.4176, 32.0618)
  line L1495 (57.4176, 32.0618) -> (57.4176, 32.4618)
  line L1496 (59.9576, 31.6618) -> (60.7476, 31.6618)
  line L1497 (60.7476, 31.6618) -> (60.7476, 31.2618)
  line L1498 (60.7476, 31.2618) -> (59.9576, 31.2618)
  line L1499 (59.9576, 31.2618) -> (59.9576, 31.6618)
  line L1500 (57.4176, 31.6618) -> (58.2076, 31.6618)
  line L1501 (58.2076, 31.6618) -> (58.2076, 31.2618)
  line L1502 (58.2076, 31.2618) -> (57.4176, 31.2618)
  line L1503 (57.4176, 31.2618) -> (57.4176, 31.6618)
  line L1504 (58.2826, 38.5368) -> (59.8826, 38.5368)
  line L1505 (59.8826, 38.5368) -> (59.8826, 37.8868)
  line L1506 (59.8826, 37.8868) -> (58.2826, 37.8868)
  line L1507 (58.2826, 37.8868) -> (58.2826, 38.5368)
  line L1508 (58.2826, 30.6368) -> (59.8826, 30.6368)
  line L1509 (59.8826, 30.6368) -> (59.8826, 29.9868)
  line L1510 (59.8826, 29.9868) -> (58.2826, 29.9868)
  line L1511 (58.2826, 29.9868) -> (58.2826, 30.6368)
  line L1512 (78.7576, 75.0368) -> (79.5476, 75.0368)
  line L1513 (79.5476, 75.0368) -> (79.5476, 74.6368)
  line L1514 (79.5476, 74.6368) -> (78.7576, 74.6368)
  line L1515 (78.7576, 74.6368) -> (78.7576, 75.0368)
  line L1516 (76.2176, 75.0368) -> (77.0076, 75.0368)
  line L1517 (77.0076, 75.0368) -> (77.0076, 74.6368)
  line L1518 (77.0076, 74.6368) -> (76.2176, 74.6368)
  line L1519 (76.2176, 74.6368) -> (76.2176, 75.0368)
  line L1520 (78.7576, 74.2368) -> (79.5476, 74.2368)
  line L1521 (79.5476, 74.2368) -> (79.5476, 73.8368)
  line L1522 (79.5476, 73.8368) -> (78.7576, 73.8368)
  line L1523 (78.7576, 73.8368) -> (78.7576, 74.2368)
  line L1524 (76.2176, 74.2368) -> (77.0076, 74.2368)
  line L1525 (77.0076, 74.2368) -> (77.0076, 73.8368)
  line L1526 (77.0076, 73.8368) -> (76.2176, 73.8368)
  line L1527 (76.2176, 73.8368) -> (76.2176, 74.2368)
  line L1528 (78.7576, 73.4368) -> (79.5476, 73.4368)
  line L1529 (79.5476, 73.4368) -> (79.5476, 73.0368)
  line L1530 (79.5476, 73.0368) -> (78.7576, 73.0368)
  line L1531 (78.7576, 73.0368) -> (78.7576, 73.4368)
  line L1532 (76.2176, 73.4368) -> (77.0076, 73.4368)
  line L1533 (77.0076, 73.4368) -> (77.0076, 73.0368)
  line L1534 (77.0076, 73.0368) -> (76.2176, 73.0368)
  line L1535 (76.2176, 73.0368) -> (76.2176, 73.4368)
  line L1536 (78.7576, 72.6368) -> (79.5476, 72.6368)
  line L1537 (79.5476, 72.6368) -> (79.5476, 72.2368)
  line L1538 (79.5476, 72.2368) -> (78.7576, 72.2368)
  line L1539 (78.7576, 72.2368) -> (78.7576, 72.6368)
  line L1540 (76.2176, 72.6368) -> (77.0076, 72.6368)
  line L1541 (77.0076, 72.6368) -> (77.0076, 72.2368)
  line L1542 (77.0076, 72.2368) -> (76.2176, 72.2368)
  line L1543 (76.2176, 72.2368) -> (76.2176, 72.6368)
  line L1544 (78.7576, 71.8368) -> (79.5476, 71.8368)
  line L1545 (79.5476, 71.8368) -> (79.5476, 71.4368)
  line L1546 (79.5476, 71.4368) -> (78.7576, 71.4368)
  line L1547 (78.7576, 71.4368) -> (78.7576, 71.8368)
  line L1548 (76.2176, 71.8368) -> (77.0076, 71.8368)
  line L1549 (77.0076, 71.8368) -> (77.0076, 71.4368)
  line L1550 (77.0076, 71.4368) -> (76.2176, 71.4368)
  line L1551 (76.2176, 71.4368) -> (76.2176, 71.8368)
  line L1552 (78.7576, 71.0368) -> (79.5476, 71.0368)
  line L1553 (79.5476, 71.0368) -> (79.5476, 70.6368)
  line L1554 (79.5476, 70.6368) -> (78.7576, 70.6368)
  line L1555 (78.7576, 70.6368) -> (78.7576, 71.0368)
  line L1556 (76.2176, 71.0368) -> (77.0076, 71.0368)
  line L1557 (77.0076, 71.0368) -> (77.0076, 70.6368)
  line L1558 (77.0076, 70.6368) -> (76.2176, 70.6368)
  line L1559 (76.2176, 70.6368) -> (76.2176, 71.0368)
  line L1560 (78.7576, 70.2368) -> (79.5476, 70.2368)
  line L1561 (79.5476, 70.2368) -> (79.5476, 69.8368)
  line L1562 (79.5476, 69.8368) -> (78.7576, 69.8368)
  line L1563 (78.7576, 69.8368) -> (78.7576, 70.2368)
  line L1564 (76.2176, 70.2368) -> (77.0076, 70.2368)
  line L1565 (77.0076, 70.2368) -> (77.0076, 69.8368)
  line L1566 (77.0076, 69.8368) -> (76.2176, 69.8368)
  line L1567 (76.2176, 69.8368) -> (76.2176, 70.2368)
  line L1568 (78.7576, 69.4368) -> (79.5476, 69.4368)
  line L1569 (79.5476, 69.4368) -> (79.5476, 69.0368)
  line L1570 (79.5476, 69.0368) -> (78.7576, 69.0368)
  line L1571 (78.7576, 69.0368) -> (78.7576, 69.4368)
  line L1572 (76.2176, 69.4368) -> (77.0076, 69.4368)
  line L1573 (77.0076, 69.4368) -> (77.0076, 69.0368)
  line L1574 (77.0076, 69.0368) -> (76.2176, 69.0368)
  line L1575 (76.2176, 69.0368) -> (76.2176, 69.4368)
  line L1576 (77.0826, 76.3118) -> (78.6826, 76.3118)
  line L1577 (78.6826, 76.3118) -> (78.6826, 75.6618)
  line L1578 (78.6826, 75.6618) -> (77.0826, 75.6618)
  line L1579 (77.0826, 75.6618) -> (77.0826, 76.3118)
  line L1580 (77.0826, 68.4118) -> (78.6826, 68.4118)
  line L1581 (78.6826, 68.4118) -> (78.6826, 67.7618)
  line L1582 (78.6826, 67.7618) -> (77.0826, 67.7618)
  line L1583 (77.0826, 67.7618) -> (77.0826, 68.4118)
  line L1584 (97.6401, 37.3368) -> (98.4301, 37.3368)
  line L1585 (98.4301, 37.3368) -> (98.4301, 36.9368)
  line L1586 (98.4301, 36.9368) -> (97.6401, 36.9368)
  line L1587 (97.6401, 36.9368) -> (97.6401, 37.3368)
  line L1588 (95.1001, 37.3368) -> (95.8901, 37.3368)
  line L1589 (95.8901, 37.3368) -> (95.8901, 36.9368)
  line L1590 (95.8901, 36.9368) -> (95.1001, 36.9368)
  line L1591 (95.1001, 36.9368) -> (95.1001, 37.3368)
  line L1592 (97.6401, 36.5368) -> (98.4301, 36.5368)
  line L1593 (98.4301, 36.5368) -> (98.4301, 36.1368)
  line L1594 (98.4301, 36.1368) -> (97.6401, 36.1368)
  line L1595 (97.6401, 36.1368) -> (97.6401, 36.5368)
  line L1596 (95.1001, 36.5368) -> (95.8901, 36.5368)
  line L1597 (95.8901, 36.5368) -> (95.8901, 36.1368)
  line L1598 (95.8901, 36.1368) -> (95.1001, 36.1368)
  line L1599 (95.1001, 36.1368) -> (95.1001, 36.5368)
  line L1600 (97.6401, 35.7368) -> (98.4301, 35.7368)
  line L1601 (98.4301, 35.7368) -> (98.4301, 35.3368)
  line L1602 (98.4301, 35.3368) -> (97.6401, 35.3368)
  line L1603 (97.6401, 35.3368) -> (97.6401, 35.7368)
  line L1604 (95.1001, 35.7368) -> (95.8901, 35.7368)
  line L1605 (95.8901, 35.7368) -> (95.8901, 35.3368)
  line L1606 (95.8901, 35.3368) -> (95.1001, 35.3368)
  line L1607 (95.1001, 35.3368) -> (95.1001, 35.7368)
  line L1608 (97.6401, 34.9368) -> (98.4301, 34.9368)
  line L1609 (98.4301, 34.9368) -> (98.4301, 34.5368)
  line L1610 (98.4301, 34.5368) -> (97.6401, 34.5368)
  line L1611 (97.6401, 34.5368) -> (97.6401, 34.9368)
  line L1612 (95.1001, 34.9368) -> (95.8901, 34.9368)
  line L1613 (95.8901, 34.9368) -> (95.8901, 34.5368)
  line L1614 (95.8901, 34.5368) -> (95.1001, 34.5368)
  line L1615 (95.1001, 34.5368) -> (95.1001, 34.9368)
  line L1616 (97.6401, 34.1368) -> (98.4301, 34.1368)
  line L1617 (98.4301, 34.1368) -> (98.4301, 33.7368)
  line L1618 (98.4301, 33.7368) -> (97.6401, 33.7368)
  line L1619 (97.6401, 33.7368) -> (97.6401, 34.1368)
  line L1620 (95.1001, 34.1368) -> (95.8901, 34.1368)
  line L1621 (95.8901, 34.1368) -> (95.8901, 33.7368)
  line L1622 (95.8901, 33.7368) -> (95.1001, 33.7368)
  line L1623 (95.1001, 33.7368) -> (95.1001, 34.1368)
  line L1624 (97.6401, 33.3368) -> (98.4301, 33.3368)
  line L1625 (98.4301, 33.3368) -> (98.4301, 32.9368)
  line L1626 (98.4301, 32.9368) -> (97.6401, 32.9368)
  line L1627 (97.6401, 32.9368) -> (97.6401, 33.3368)
  line L1628 (95.1001, 33.3368) -> (95.8901, 33.3368)
  line L1629 (95.8901, 33.3368) -> (95.8901, 32.9368)
  line L1630 (95.8901, 32.9368) -> (95.1001, 32.9368)
  line L1631 (95.1001, 32.9368) -> (95.1001, 33.3368)
  line L1632 (97.6401, 32.5368) -> (98.4301, 32.5368)
  line L1633 (98.4301, 32.5368) -> (98.4301, 32.1368)
  line L1634 (98.4301, 32.1368) -> (97.6401, 32.1368)
  line L1635 (97.6401, 32.1368) -> (97.6401, 32.5368)
  line L1636 (95.1001, 32.5368) -> (95.8901, 32.5368)
  line L1637 (95.8901, 32.5368) -> (95.8901, 32.1368)
  line L1638 (95.8901, 32.1368) -> (95.1001, 32.1368)
  line L1639 (95.1001, 32.1368) -> (95.1001, 32.5368)
  line L1640 (97.6401, 31.7368) -> (98.4301, 31.7368)
  line L1641 (98.4301, 31.7368) -> (98.4301, 31.3368)
  line L1642 (98.4301, 31.3368) -> (97.6401, 31.3368)
  line L1643 (97.6401, 31.3368) -> (97.6401, 31.7368)
  line L1644 (95.1001, 31.7368) -> (95.8901, 31.7368)
  line L1645 (95.8901, 31.7368) -> (95.8901, 31.3368)
  line L1646 (95.8901, 31.3368) -> (95.1001, 31.3368)
  line L1647 (95.1001, 31.3368) -> (95.1001, 31.7368)
  line L1648 (95.9651, 38.6118) -> (97.5651, 38.6118)
  line L1649 (97.5651, 38.6118) -> (97.5651, 37.9618)
  line L1650 (97.5651, 37.9618) -> (95.9651, 37.9618)
  line L1651 (95.9651, 37.9618) -> (95.9651, 38.6118)
  line L1652 (95.9651, 30.7118) -> (97.5651, 30.7118)
  line L1653 (97.5651, 30.7118) -> (97.5651, 30.0618)
  line L1654 (97.5651, 30.0618) -> (95.9651, 30.0618)
  line L1655 (95.9651, 30.0618) -> (95.9651, 30.7118)
  line L1656 (20.5126, 12.7618) -> (19.7226, 12.7618)
  line L1657 (19.7226, 12.7618) -> (19.7226, 13.1618)
  line L1658 (19.7226, 13.1618) -> (20.5126, 13.1618)
  line L1659 (20.5126, 13.1618) -> (20.5126, 12.7618)
  line L1660 (23.0526, 12.7618) -> (22.2626, 12.7618)
  line L1661 (22.2626, 12.7618) -> (22.2626, 13.1618)
  line L1662 (22.2626, 13.1618) -> (23.0526, 13.1618)
  line L1663 (23.0526, 13.1618) -> (23.0526, 12.7618)
  line L1664 (20.5126, 13.5618) -> (19.7226, 13.5618)
  line L1665 (19.7226, 13.5618) -> (19.7226, 13.9618)
  line L1666 (19.7226, 13.9618) -> (20.5126, 13.9618)
  line L1667 (20.5126, 13.9618) -> (20.5126, 13.5618)
  line L1668 (23.0526, 13.5618) -> (22.2626, 13.5618)
  line L1669 (22.2626, 13.5618) -> (22.2626, 13.9618)
  line L1670 (22.2626, 13.9618) -> (23.0526, 13.9618)
  line L1671 (23.0526, 13.9618) -> (23.0526, 13.5618)
  line L1672 (20.5126, 14.3618) -> (19.7226, 14.3618)
  line L1673 (19.7226, 14.3618) -> (19.7226, 14.7618)
  line L1674 (19.7226, 14.7618) -> (20.5126, 14.7618)
  line L1675 (20.5126, 14.7618) -> (20.5126, 14.3618)
  line L1676 (23.0526, 14.3618) -> (22.2626, 14.3618)
  line L1677 (22.2626, 14.3618) -> (22.2626, 14.7618)
  line L1678 (22.2626, 14.7618) -> (23.0526, 14.7618)
  line L1679 (23.0526, 14.7618) -> (23.0526, 14.3618)
  line L1680 (20.5126, 15.1618) -> (19.7226, 15.1618)
  line L1681 (19.7226, 15.1618) -> (19.7226, 15.5618)
  line L1682 (19.7226, 15.5618) -> (20.5126, 15.5618)
  line L1683 (20.5126, 15.5618) -> (20.5126, 15.1618)
  line L1684 (23.0526, 15.1618) -> (22.2626, 15.1618)
  line L1685 (22.2626, 15.1618) -> (22.2626, 15.5618)
  line L1686 (22.2626, 15.5618) -> (23.0526, 15.5618)
  line L1687 (23.0526, 15.5618) -> (23.0526, 15.1618)
  line L1688 (20.5126, 15.9618) -> (19.7226, 15.9618)
  line L1689 (19.7226, 15.9618) -> (19.7226, 16.3618)
  line L1690 (19.7226, 16.3618) -> (20.5126, 16.3618)
  line L1691 (20.5126, 16.3618) -> (20.5126, 15.9618)
  line L1692 (23.0526, 15.9618) -> (22.2626, 15.9618)
  line L1693 (22.2626, 15.9618) -> (22.2626, 16.3618)
  line L1694 (22.2626, 16.3618) -> (23.0526, 16.3618)
  line L1695 (23.0526, 16.3618) -> (23.0526, 15.9618)
  line L1696 (20.5126, 16.7618) -> (19.7226, 16.7618)
  line L1697 (19.7226, 16.7618) -> (19.7226, 17.1618)
  line L1698 (19.7226, 17.1618) -> (20.5126, 17.1618)
  line L1699 (20.5126, 17.1618) -> (20.5126, 16.7618)
  line L1700 (23.0526, 16.7618) -> (22.2626, 16.7618)
  line L1701 (22.2626, 16.7618) -> (22.2626, 17.1618)
  line L1702 (22.2626, 17.1618) -> (23.0526, 17.1618)
  line L1703 (23.0526, 17.1618) -> (23.0526, 16.7618)
  line L1704 (20.5126, 17.5618) -> (19.7226, 17.5618)
  line L1705 (19.7226, 17.5618) -> (19.7226, 17.9618)
  line L1706 (19.7226, 17.9618) -> (20.5126, 17.9618)
  line L1707 (20.5126, 17.9618) -> (20.5126, 17.5618)
  line L1708 (23.0526, 17.5618) -> (22.2626, 17.5618)
  line L1709 (22.2626, 17.5618) -> (22.2626, 17.9618)
  line L1710 (22.2626, 17.9618) -> (23.0526, 17.9618)
  line L1711 (23.0526, 17.9618) -> (23.0526, 17.5618)
  line L1712 (20.5126, 18.3618) -> (19.7226, 18.3618)
  line L1713 (19.7226, 18.3618) -> (19.7226, 18.7618)
  line L1714 (19.7226, 18.7618) -> (20.5126, 18.7618)
  line L1715 (20.5126, 18.7618) -> (20.5126, 18.3618)
  line L1716 (23.0526, 18.3618) -> (22.2626, 18.3618)
  line L1717 (22.2626, 18.3618) -> (22.2626, 18.7618)
  line L1718 (22.2626, 18.7618) -> (23.0526, 18.7618)
  line L1719 (23.0526, 18.7618) -> (23.0526, 18.3618)
  line L1720 (22.1876, 11.4868) -> (20.5876, 11.4868)
  line L1721 (20.5876, 11.4868) -> (20.5876, 12.1368)
  line L1722 (20.5876, 12.1368) -> (22.1876, 12.1368)
  line L1723 (22.1876, 12.1368) -> (22.1876, 11.4868)
  line L1724 (22.1876, 19.3868) -> (20.5876, 19.3868)
  line L1725 (20.5876, 19.3868) -> (20.5876, 20.0368)
  line L1726 (20.5876, 20.0368) -> (22.1876, 20.0368)
  line L1727 (22.1876, 20.0368) -> (22.1876, 19.3868)
  line L1728 (132.892, 0.0262) -> (0.05, 0.0262)
  line L1729 (0.05, 0.0262) -> (0.05, 90.8566)
  line L1730 (0.05, 90.8566) -> (132.892, 90.8566)
  line L1731 (132.892, 90.8566) -> (132.892, 0.0262)
  point P0 (0, 0)
  point P1 (0.05, 0.0262)
  constraints: 3464 end point
extrude "Extrusion1" add sketch "Skizze5" along normal blind 1